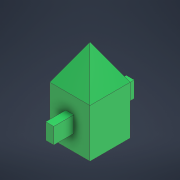
# Autodesk Inventor part: 110033226_ipt_21_柵欄
Saved by Autodesk Inventor 2022 (Build 260153000, 153)
## iProperties
Created: 2022-06-23
Part Number: 110033226_ipt_21_柵欄
Material: 一般
Document SubType Name: Modeling
Designer: User
Density: 1 g/cm^3
Appearance: 預設
Author: User
Autodesk Inventor part; units mm, degrees
ref_plane "YZ Plane" through (0, 0, 0) normal (1, 0, 0) x (0, 1, 0)
ref_plane "XZ Plane" through (0, 0, 0) normal (0, 1, 0) x (-1, 0, 0)
ref_plane "XY Plane" through (0, 0, 0) normal (0, 0, 1) x (1, 0, 0)
sketch "草圖1" plane through (0, 0, 0) normal (0, 1, 0) x (-1, 0, 0)
  line L0 (2.5, 2.5) -> (-2.5, 2.5)
  line L1 (-2.5, 2.5) -> (-2.5, -2.5)
  line L2 (-2.5, -2.5) -> (2.5, -2.5)
  line L3 (2.5, -2.5) -> (2.5, 2.5)
  circle A0 centre (0, 0) radius 1.7
  point P0 (2.5, 0)
  point P1 (0, -2.5)
  dimension "d0" = 5
  dimension "d1" = 5
  dimension "d2" = 3.4
  constraints: 8 end point, 2 midpoint, 2 parallel, 1 centre point, 1 coincident, 1 horizontal, 1 horizontal alignment, 1 perpendicular, 1 vertical alignment
  measures "d0" distance of L2.end L1.end
  measures "d1" distance of L1.end L0.end
  measures "d2" diameter of A0
extrude "擠出1" add sketch "草圖1" along normal blind 6 contours L3 L2 L1 L0 | A0
extrude "擠出2" cut sketch "草圖1" along normal blind 1.5 contours A0
sketch "草圖2" plane through (0, 6, 0) normal (0, 1, 0) x (1, 0, 0)
  line L0 (2.5, -2.5) -> (2.5, 2.5) projected
  line L1 (2.5, 2.5) -> (-2.5, 2.5) projected
  line L2 (-2.5, 2.5) -> (-2.5, -2.5) projected
  line L3 (-2.5, -2.5) -> (2.5, -2.5) projected
  point P0 (0, 0)
extrude "擠出3" add sketch "草圖2" along normal blind 15 draft -30
sketch "草圖3" plane through (2.5, 0, -2.5) normal (0, 0, -1) x (-1, 0, 0)
  line L0 (0, 0) -> (5, 0) projected
  line L1 (5, 0) -> (5, 6) projected
  line L2 (0, 6) -> (5, 6) projected
  line L3 (0, 0) -> (0, 6) projected
  line L4 (3, 4) -> (3, 2)
  line L5 (3, 2) -> (2, 2)
  line L6 (2, 2) -> (2, 4)
  line L7 (2, 4) -> (3, 4)
  point P0 (2.5, 0)
  dimension "d9" = 2
  constraints: 8 end point, 3 other
  measures "d9" distance between parallel lines of L2 L7
extrude "擠出4" add sketch "草圖3" along normal blind 2.5 contours L4 L5 L6 L7
mirror "鏡射1" about plane through (0, 0, 0) normal (0, 0, 1) of "擠出4"
